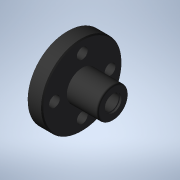
# Autodesk Inventor part: C-LHFR5
Saved by Autodesk Inventor 2021 (Build 250183000, 183)
## iProperties
Created: 2025-08-07
Part Number: C-LHFR5
Material: Generic
Catalog Web Link: www.cadenas.de
Description: C-LHFR, C-LHFS, C-LHFC, C-LHFRM, C-LHFSM, C-LHFCM,C-LHFCF-N,C-LHFCMF-N-Flanged Linear Bushings - Standard - C-VALUE Single Type
Vendor: MISUMI
Document SubType Name: Modeling
Designer: psAdmin
Manufacturer: MISUMI
Mass: 2.70355 g
Surface Area: 21.9703 cm^2
Volume: 2.70355 cm^3
Density: 1 g/cm^3
Appearance: PSOLRGB-175-175-175
Category: PARTsolutions
Company: MISUMI
Title: C-LHFR5
Author: Cadenas PARTsolutions
Comments: Flanged Linear Bushings - Standard - C-VALUE Single Type
PSOL_IDENT_0: {$CADENAS_DATA/23d-libs/misumi/metric/04_linear_bushings/c_lhfr.prj},226 {VTYP=3D},{NB=C-LHFR5},{LIN
PSOL_IDENT_1: A=C-LHFR5},{NN=C-LHFR, C-LHFS, C-LHFC, C-LHFRM, C-LHFSM, C-LHFCM,C-LHFCF-N,C-LHFCMF-N},{DATE=16.08.2
PSOL_IDENT_2: 023 02:43:51},{GEOMDATE=03.08.2023 03:48:35},{VERSION=},{LINEID=40},{WBVAR=SS,TS,ST},{WBNUMERIC=}  {
PSOL_IDENT_3: NB=C-LHFR5},{LINA=C-LHFR5},{KT=DUMMY},{PN=C-LHFR5},{TYPE=C-LHFR},{SS=S},{SSALG='S','Standard Specifi
PSOL_IDENT_4: cations','HT','High Temperature Specification'},{TS=R},{TSALG='R', 'Round Flange', 'S', 'Square Flan
PSOL_IDENT_5: ge', 'C', '2 - Flats Flange'},{ST=},{STALG='', '-'},{DDRR=5},{D=10},{L=15},{H=26},{T=5},{DD=3.5},{DD
PSOL_IDENT_6: 1=6.0},{TT=3.1},{PCD=18},{PCDFX=18},{W=0},{WFX=21},{F=0},{FFX=0},{A=0},{AFX=18},{K=0},{KFX=16},{BR=4
PSOL_IDENT_7: },{TIFF=1},{R=0.5},{C=0.35},{DD2=5.4},{DD3=5.8},{Y=0.4},{Z=0.30}
NB: C-LHFR5
NN: C-LHFR, C-LHFS, C-LHFC, C-LHFRM, C-LHFSM, C-LHFCM,C-LHFCF-N,C-LHFCMF-N
NT: Flanged Linear Bushings - Standard - C-VALUE Single Type
NBSYN: $PN.
LINA: C-LHFR5
CATALOG: Misumi
PN: C-LHFR5
TYPE: C-LHFR
SS: Standard Specifications
TS: Round Flange
ST: -
DDRR: 5
D: 10
L: 15
H: 26
T: 5
DD: 3.5
DD1: 6
TT: 3.1
PCD: 18
W: 0
F: 0
A: 0
K: 0
SUPPLIER: MISUMI
ARTICLENO: C-LHFR5
BOMINFO: C-LHFR5
CREATOR: CADENAS GmbH
Autodesk Inventor part; units mm, degrees
sketch "Sketch_1" plane through (0, 0, 0) normal (0, 0, 1) x (1, 0, 0)
  line L0 (15, 0) -> (0, 0)
  line L1 (0, 2.7) -> (0.4, 2.7)
  line L2 (0.4, 2.7) -> (0.4, 2.9)
  line L3 (0.4, 2.9) -> (0.7, 2.9)
  line L4 (0.7, 2.9) -> (0.7, 2.5)
  line L5 (0.7, 2.5) -> (14.3, 2.5)
  line L6 (14.3, 2.5) -> (14.3, 2.9)
  line L7 (14.3, 2.9) -> (14.6, 2.9)
  line L8 (14.6, 2.9) -> (14.6, 2.7)
  line L9 (14.6, 2.7) -> (15, 2.7)
  line L10 (15, 2.7) -> (15, 4.5)
  arc A0 (15, 4.5) -> (14.5, 5) centre (14.5, 4.5) ccw
  line L11 (14.5, 5) -> (5, 5)
  line L12 (5, 5) -> (5, 12.65)
  line L13 (5, 12.65) -> (4.65, 13)
  line L14 (4.65, 13) -> (0.35, 13)
  line L15 (0.35, 13) -> (0, 12.65)
  line L16 (0, 12.65) -> (0, 2.7)
  constraints: 34 end point, 2 point on circle, 1 centre point
revolve "Revolution1" add sketch "Sketch_1" angle 360 about axis through (15, 0, 0) along (1, 0, 0)
sketch "Sketch2" plane through (0, 0, 0) normal (-1, 0, 0) x (0, 0, 1)
  point P0 (0, 9)
hole "Hole1" at (0, 9, 0) direction (1, 0, 0) diameter 3.5 depth 5 counterbore diameter 6 counterbore depth 3.1
sketch "Sketch3" plane through (0, 0, 0) normal (-1, 0, 0) x (0, 0, 1)
  point P0 (0, -9)
hole "Hole2" at (0, -9, 0) direction (1, 0, 0) diameter 3.5 depth 5 counterbore diameter 6 counterbore depth 3.1
sketch "Sketch4" plane through (0, 0, 0) normal (-1, 0, 0) x (0, 0, 1)
  point P0 (-9, 0)
hole "Hole3" at (0, 0, -9) direction (1, 0, 0) diameter 3.5 depth 5 counterbore diameter 6 counterbore depth 3.1
sketch "Sketch5" plane through (0, 0, 0) normal (-1, 0, 0) x (0, 0, 1)
  point P0 (9, 0)
hole "Hole4" at (0, 0, 9) direction (1, 0, 0) diameter 3.5 depth 5 counterbore diameter 6 counterbore depth 3.1
ref_plane "Combination_Module_XY" through (0, 0, 0) normal (1, 0, 0) x (0, 0, -1)
ref_plane "Combination_Module_YZ" through (0, 0, 0) normal (0, 0, -1) x (0, 1, 0)
ref_plane "Combination_Module_ZX" through (0, 0, 0) normal (0, 1, 0) x (1, 0, 0)
body "Solid1"
